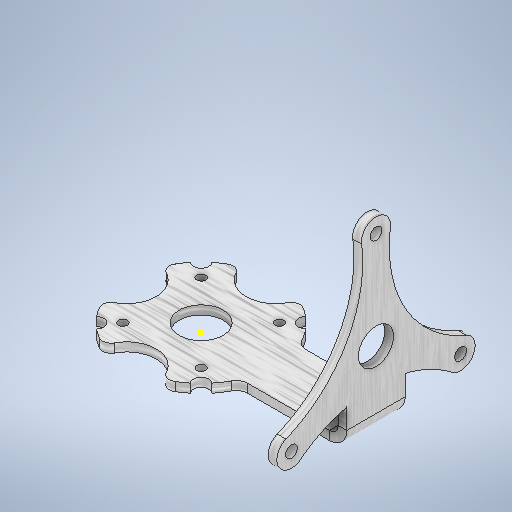
# Autodesk Inventor part: J4_J5_CONNECTOR
Saved by Autodesk Inventor 2025.4 (Build 294407000, 407)
## iProperties
Created: 2026-06-09
Part Number: J4_J5_CONNECTOR
Material: 铝 5052
Document SubType Name: Sheet Metal
Designer: Admin
Density: 2.68 g/cm^3
Sheet Metal Rule: 默认_mm
Appearance: 缎光 - 强拉丝
Mass: 24.5757 g
Surface Area: 79.7822 cm^2
Volume: 9.17003 cm^3
Author: Admin
Autodesk Inventor part; units mm, degrees
ref_plane "YZ Plane" through (0, 0, 0) normal (1, 0, 0) x (0, 1, 0)
ref_plane "XZ Plane" through (0, 0, 0) normal (0, 1, 0) x (-1, 0, 0)
ref_plane "XY Plane" through (0, 0, 0) normal (0, 0, 1) x (1, 0, 0)
sketch "草图1" plane through (0, 0, 0) normal (0, 1, 0) x (-1, 0, 0)
  point P0 (0, 0)
sketch "草图2" plane through (0, 0, 0) normal (0, 1, 0) x (-1, 0, 0)
  circle A0 centre (0, 0) radius 25.5
  dimension "d0" = 51
  measures "d0" diameter of A0
extrude "平板1" add sketch "草图2" along normal blind 3
sketch "草图4" plane through (0, 0, 0) normal (0, -1, 0) x (1, 0, 0)
  line L0 (-7.9097, 24.2233) -> (-8.2692, 24.0903)
  line L1 (-4.4157, 25.11) -> (-4.7246, 25.0488)
  circle A0 centre (13.435, -13.435) radius 1.35
  circle A1 centre (-13.435, -13.435) radius 1.35
  circle A2 centre (-13.435, 13.435) radius 1.35
  circle A3 centre (13.435, 13.435) radius 1.35
  arc A4 (-16.1014, -19.7736) -> (-19.7736, -16.1014) centre (-18.0312, -18.0312) ccw
  arc A5 (19.7736, -16.1014) -> (16.1014, -19.7736) centre (18.0312, -18.0312) ccw
  arc A6 (16.1014, 19.7736) -> (19.7736, 16.1014) centre (18.0312, 18.0312) ccw
  arc A7 (-19.7736, 16.1014) -> (-16.1014, 19.7736) centre (-18.0312, 18.0312) ccw
  circle A8 centre (0, 0) radius 25.5
  arc A9 (9.8059, -23.5392) -> (-9.8059, -23.5392) centre (0, -25.5) ccw
  arc A10 (-23.5392, -9.8059) -> (-23.5392, 9.8059) centre (-25.5, 0) ccw
  circle A11 centre (0, 0) radius 25.5 projected
  arc A12 (-9.8059, 23.5392) -> (9.8059, 23.5392) centre (0, 25.5) ccw
  dimension "d4" = 20
  constraints: 14 point on circle, 11 centre point, 4 end point, 2 equal radius, 21 other
  measures "d4" diameter of A9
extrude "拉伸2" cut sketch "草图4" against normal blind 10 contours A0 | A1 | A2 | A3 | A8 A4 | A9 A8 | A8 A10 | A5 A8 | A8 A7 | A8 A12 | A6 A8
fillet "圆角1" radius 3 6 edges at (-9.8059, 1.5, -23.5392) (9.8059, 1.5, -23.5392) (-23.5392, 1.5, 9.8059) (-23.5392, 1.5, -9.8059) (9.8059, 1.5, 23.5392) (-9.8059, 1.5, 23.5392)
sketch "草图5" plane through (0, 0, 0) normal (0, -1, 0) x (1, 0, 0)
  line L0 (0, 10) -> (57, 10)
  line L1 (57, 10) -> (57, -10)
  line L2 (57, -10) -> (0, -10)
  line L3 (0, -10) -> (0, 10)
  line L4 (0, 50.3161) -> (0, -50.0414)
  point P0 (0, 0)
  dimension "d8" = 20
  dimension "d9" = 10
  dimension "d10" = 57
  measures "d8" distance of L0.end L1.end
  measures "d9" distance from line of point (0, 0) L2
  measures "d10" distance of L0.start L0.end
sheet face with bend "平板2" sketch "草图5" thickness 3 toward (0, 1, 0) bend radius 3
bend "折弯1"
fillet "圆角2" radius 4 2 edges at (23.4574, 1.5, -10) (23.4574, 1.5, 10)
sketch "草图6" plane through (0, 0, 0) normal (0, -1, 0) x (1, 0, 0)
  point P0 (0, 0)
  point P1 (0, 0)
  constraints: 1 coincident
hole "孔1" at (0, 0, 0) direction (0, 1, 0) diameter 15 end through all
sketch "草图7" plane through (60, 0, -10) normal (-1, 0, 0) x (0, -1, 0)
  line L0 (0, 20) -> (0, 0)
  line L1 (0, 0) -> (-15, 0)
  line L2 (-15, 0) -> (-15, 20)
  line L3 (-15, 20) -> (0, 20)
  constraints: 8 end point
edge flange "凸缘1" height 15 angle 90 thickness 3 bend radius 3 thickness toward (-1, 0, 0) relief tear relief width 3 relief depth 1.5 edges at (57, 3, 0) wall of the first edge with corners at (60, 0, 10) (60, 0, -10) (60, 15, -10) (60, 15, 10)
bend "折弯2"
corner "拐角1"
sketch "草图9" plane through (0, 0, 0) normal (0, -1, 0) x (1, 0, 0)
  circle A0 centre (13.435, 13.435) radius 1.35 projected
  circle A1 centre (13.435, -13.435) radius 1.35 projected
  circle A2 centre (-13.435, -13.435) radius 1.35 projected
  circle A3 centre (-13.435, 13.435) radius 1.35 projected
  point P0 (0, 0)
hole "孔2" at (13.435, 0, 13.435) at (13.435, 0, -13.435) at (-13.435, 0, -13.435) at (-13.435, 0, 13.435) direction (0, 1, 0) diameter 3 end through all
sketch "草图12" plane through (0, 0, 0) normal (0, -1, 0) x (1, 0, 0)
  line L0 (54, -10) -> (54, 10) projected
  line L1 (54, 10) -> (25.9663, 10) projected
  point P0 (0, 0)
  point P1 (45, -5)
  point P2 (45, 5)
  dimension "d64" = 10
  dimension "d65" = 9
  dimension "d66" = 5
  constraints: 1 vertical alignment
  measures "d64" distance of point (45, 5) point (45, -5)
  measures "d65" distance from line of L0 point (45, 5)
  measures "d66" distance from line of L1 point (45, 5)
hole "孔3" at (45, 0, -5) at (45, 0, 5) direction (0, 1, 0) diameter 3 end through all
sketch "草图21" plane through (60, 15, 10) normal (1, 0, 0) x (0, 0, -1)
  circle A0 centre (10, 11) radius 33.5
  circle A1 centre (10, 44.5) radius 5
  circle A2 centre (-19.0119, -5.75) radius 5
  circle A3 centre (39.0119, -5.75) radius 5
  circle A4 centre (57.0777, 38.1803) radius 42.5
  circle A5 centre (-37.0777, 38.1803) radius 42.5
  circle A6 centre (10, -43.3607) radius 42.5
  circle A7 centre (10, 11) radius 6
  point P0 (10, -15)
  point P1 (-15.958, -9.709)
  point P2 (35.958, -9.709)
  point P3 (40.9135, -1.1258)
  point P4 (14.9555, 43.8348)
  point P5 (5.0445, 43.8348)
  point P6 (-20.9135, -1.1258)
  dimension "d112" = 67
  dimension "d113" = 10
  dimension "d116" = 360
  dimension "d118" = 85
  dimension "d131" = 12
  measures "d113" diameter of A1
  measures "d118" diameter of A4
  measures "d131" diameter of A7
sheet face with bend "平板7" sketch "草图21" thickness 3 toward (-1, 0, 0) bend radius 3 contours A1 A0 | A0 A1 | A4 A3 A6 A2 A5 A1 | A3 A0 | A0 A3 | A2 A0 | A2 A0
bend "折弯7"
sketch "草图22" plane through (60, 6, 10) normal (1, 0, 0) x (0, 0, -1)
  arc A0 (36.1869, -0.8925) -> (41.8368, 7.3925) centre (39.0119, 3.25) ccw
  arc A1 (15, 53.1248) -> (5, 53.8752) centre (10, 53.5) ccw
  arc A2 (-21.1869, 7.7677) -> (-16.8368, -1.2677) centre (-19.0119, 3.25) ccw
  point P0 (10, -6)
  constraints: 6 point on circle, 3 centre point, 12 other
hole "孔6" at (60, 59.5, 0) at (60, 9.25, -29.0119) at (60, 9.25, 29.0119) direction (-1, 0, 0) diameter 4 end through all
equation "\"d22\" = 厚度"
equation "\"d1\" = 厚度"
equation "\"d11\" = 折弯半径"
equation "\"d12\" = 折弯释压宽度"
equation "\"d13\" = 折弯释压深度"
equation "\"d14\" = 最小余量"
equation "\"d15\" = 过渡半径"
equation "\"d24\" = 折弯释压宽度"
equation "\"d25\" = 折弯释压深度"
equation "\"d26\" = 最小余量"
equation "\"d27\" = 过渡半径"
equation "\"d30\" = 折弯半径"
equation "\"d31\" = 拐角释压尺寸"
equation "\"d32\" = 间隙大小"
equation "\"d33\" = Jacobi半径尺寸"
equation "\"折弯半径\" = 厚度"
equation "\"折弯释压宽度\" = 厚度"
equation "\"折弯释压深度\" = 0.5 * 厚度"
equation "\"拐角释压尺寸\" = 4 * 厚度"
equation "\"最小余量\" = 2 * 厚度"
equation "\"过渡半径\" = 折弯半径"
equation "\"Jacobi半径尺寸\" = 折弯半径"
equation "\"间隙大小\" = 厚度"
equation "\"厚度\" = 3"
